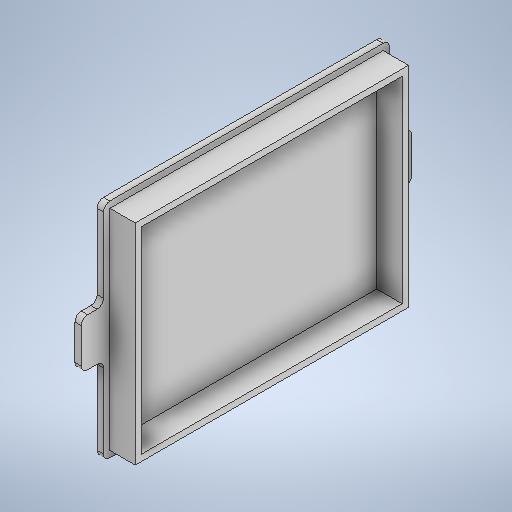
# Autodesk Inventor part: Couv
Saved by Autodesk Inventor 2025 (Build 290162000, 162)
## iProperties
Created: 2024-05-29
Part Number: Couv
Material: Générique
Document SubType Name: Modeling
Designer: luc4s
Density: 1 g/cm^3
Appearance: Par défaut
Author: luc4s
Autodesk Inventor part; units mm, degrees
ref_plane "YZ Plane" through (0, 0, 0) normal (1, 0, 0) x (0, 1, 0)
ref_plane "XZ Plane" through (0, 0, 0) normal (0, 1, 0) x (-1, 0, 0)
ref_plane "XY Plane" through (0, 0, 0) normal (0, 0, 1) x (1, 0, 0)
sketch "Esquisse1" plane through (0, 0, 0) normal (1, 0, 0) x (0, 1, 0)
  line L0 (35, 45) -> (-35, 45)
  line L1 (-35, 45) -> (-35, -45)
  line L2 (-35, -45) -> (35, -45)
  line L3 (35, -45) -> (35, 45)
  line L4 (26.5459, 0) -> (-33.52, 0) construction
  line L5 (0, 24.5499) -> (0, -29.9835) construction
  point P0 (0, 0)
  dimension "d0" = 90
  dimension "d1" = 70
  constraints: 12 end point, 2 horizontal, 2 parallel, 2 perpendicular, 2 point on line, 2 other
  measures "d0" distance of L2.end L0.start
  measures "d1" distance of L0.start L0.end
extrude "Extrusion1" add sketch "Esquisse1" along normal blind 2
sketch "Esquisse2" plane through (2, 0, 0) normal (1, 0, 0) x (0, 0, -1)
  line L0 (-43, 33) -> (43, 33)
  line L1 (43, 33) -> (43, -33)
  line L2 (43, -33) -> (-43, -33)
  line L3 (-43, -33) -> (-43, 33)
  line L4 (-41, 31) -> (41, 31)
  line L5 (41, 31) -> (41, -31)
  line L6 (41, -31) -> (-41, -31)
  line L7 (-41, -31) -> (-41, 31)
  line L8 (45, 35) -> (-45, 35) projected
  line L9 (-45, 35) -> (-45, -35) projected
  line L10 (-45, -35) -> (45, -35) projected
  line L11 (45, -35) -> (45, 35) projected
  dimension "d4" = 2
  dimension "d5" = 2
  dimension "d6" = 2
  dimension "d7" = 2
  dimension "d8" = 2
  dimension "d9" = 2
  dimension "d10" = 2
  dimension "d11" = 2
  constraints: 16 end point, 4 parallel, 2 horizontal, 2 perpendicular
  measures "d4" distance between parallel lines of L0 L8
  measures "d5" distance between parallel lines of L9 L3
  measures "d6" distance between parallel lines of L10 L2
  measures "d7" distance between parallel lines of L11 L1
  measures "d8" distance between parallel lines of L0 L4
  measures "d9" distance between parallel lines of L1 L5
  measures "d10" distance between parallel lines of L2 L6
  measures "d11" distance between parallel lines of L3 L7
extrude "Extrusion2" add sketch "Esquisse2" along normal blind 8 contours L0 L1 L2 L3
sketch "Esquisse3" plane through (0, -35, -45) normal (0, 0, -1) x (-1, 0, 0)
  point P0 (0, 35)
sketch "Esquisse4" plane through (2, 0, 0) normal (1, 0, 0) x (0, 0, -1)
  line L0 (45, -35) -> (45, 35) projected
  line L1 (45, -7.5) -> (52, -7.5)
  line L2 (52, -7.5) -> (52, 7.5)
  line L3 (52, 7.5) -> (45, 7.5)
  line L4 (45, 7.5) -> (45, -7.5)
  point P0 (0, 0)
  dimension "d14" = 15
  dimension "d15" = 7
  dimension "d16" = 27.5
  constraints: 8 end point, 2 parallel, 1 horizontal, 1 perpendicular, 1 point on line
  measures "d14" distance between parallel lines of L3 L1
  measures "d15" distance of L2.end L3.end
  measures "d16" distance from line of L1 L0.start
extrude "Extrusion3" add sketch "Esquisse4" against normal blind 2
fillet "Congé1" radius 2 5 edges at (1, 35, -45) (1, 7.5, -52) (1, -7.5, -52) (1, 7.5, -45) (1, -35, -45)
fillet "Congé2" radius 2 1 edges at (1, -7.5, -45)
mirror "Mise en miroir1" about plane through (0, 0, 0) normal (0, 0, 1) of "Extrusion3"
fillet "Congé3" radius 2 5 edges at (1, -35, 45) (1, -7.5, 45) (1, -7.5, 52) (1, 7.5, 52) (1, 35, 45)
fillet "Congé4" radius 2 1 edges at (1, 7.5, 45)
sketch "Esquisse5" plane through (0, 0, 0) normal (-1, 0, 0) x (0, 0, 1)
  circle A0 centre (-48, 3.5) radius 1.75
  line L0 (-52, 5.5) -> (-52, -5.5) projected
  line L1 (-47, 7.5) -> (-50, 7.5) projected
  point P0 (0, 0)
  dimension "d23" = 3.5
  dimension "d24" = 4
  dimension "d25" = 4
  constraints: 1 centre point
  measures "d23" diameter of A0
  measures "d24" distance from line of L0 A0.centre
  measures "d25" distance from line of L1 A0.centre
extrude "Extrusion4" cut sketch "Esquisse5" against normal blind 2
mirror "Mise en miroir2" about plane through (0, 0, 0) normal (0, 1, 0) of "Extrusion4"
